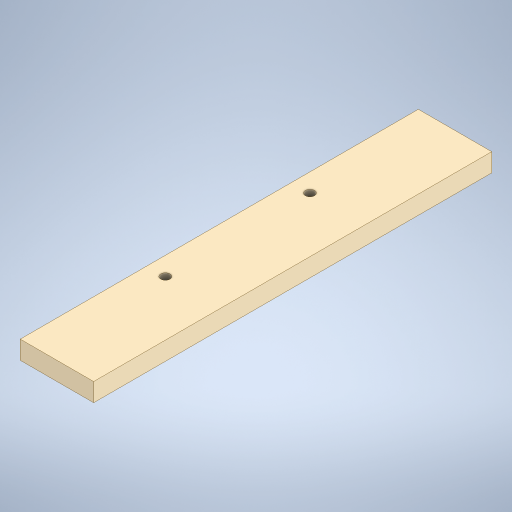
# Autodesk Inventor part: Wood-8
Saved by Autodesk Inventor 2024 (Build 280153000, 153)
## iProperties
Created: 2024-03-21
Part Number: Wood-8
Material: Generic
Document SubType Name: Modeling
Designer: anyangoe
Density: 1 g/cm^3
Appearance: Default
Author: anyangoe
Autodesk Inventor part; units mm, degrees
ref_plane "YZ Plane" through (0, 0, 0) normal (1, 0, 0) x (0, 1, 0)
ref_plane "XZ Plane" through (0, 0, 0) normal (0, 1, 0) x (-1, 0, 0)
ref_plane "XY Plane" through (0, 0, 0) normal (0, 0, 1) x (1, 0, 0)
sketch "Sketch1" plane through (0, 0, 0) normal (0, 1, 0) x (-1, 0, 0)
  line L0 (0, 0) -> (50.8, 0)
  line L1 (50.8, 0) -> (50.8, -275.4)
  line L2 (50.8, -275.4) -> (0, -275.4)
  line L3 (0, -275.4) -> (0, 0)
  dimension "d0" = 50.8
  dimension "d1" = 275.4
  constraints: 8 end point, 2 parallel, 1 horizontal, 1 perpendicular
  measures "d0" distance of L0.start L0.end
  measures "d1" distance of L2.end L0.start
extrude "Extrusion1" add sketch "Sketch1" along normal blind 12.7
sketch "Sketch2" plane through (0, 12.7, 0) normal (0, 1, 0) x (1, 0, 0)
  circle A0 centre (-38.1, 87.7) radius 3.175
  circle A1 centre (-38.1, 187.7) radius 3.175
  line L0 (-50.8, 0) -> (0, 0) projected
  line L1 (0, 0) -> (0, 275.4) projected
  dimension "d4" = 87.7
  dimension "d5" = 100
  dimension "d6" = 6.35
  dimension "d7" = 38.1
  constraints: 2 centre point, 1 equal radius, 1 vertical alignment
  measures "d4" distance from line of L0 A0.centre
  measures "d5" distance of A1.centre A0.centre
  measures "d6" diameter of A1
  measures "d7" distance from line of L1 A1.centre
extrude "Extrusion2" cut sketch "Sketch2" against normal blind 12.7
body "Solid1"
